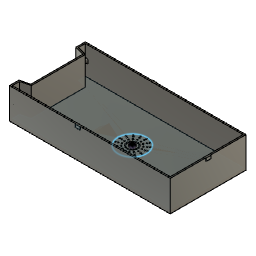
coolingpadbox v18 (Autodesk Fusion 360 design; units mm, degrees)
Autodesk Fusion 360 part; units mm, degrees
sketch "Sketch1" plane through (0, 0, 0) normal (1, 0, 0) x (0, 1, 0)
sketch "Sketch2" plane through (0, 0, 0) normal (0, 1, 0) x (1, 0, 0)
sketch "Sketch3" plane through (0, 0, 0) normal (0, 0, 1) x (1, 0, 0)
  line L0 (-89.6492, -40) -> (80, -40)
  line L1 (80, -40) -> (80, 40)
  line L2 (80, 40) -> (-89.6492, 40)
  line L3 (-89.6492, 40) -> (-89.6492, 30)
  line L4 (-89.6492, -40) -> (-89.6492, -30)
  line L5 (-89.6492, -40) -> (-79.6492, -40)
  line L6 (-79.6492, 27.5) -> (-79.6492, -27.5)
  line L7 (-79.6492, 27.5) -> (-89.6492, 30)
  line L8 (-89.6492, -30) -> (-79.6492, -27.5)
  constraint horizontal L0
  constraint perpendicular L0 L1
  constraint perpendicular L1 L2
  constraint coincident L0 L5.end
extrude "Extrude1" add sketch "Sketch3" along normal blind 2.5
sketch "Sketch4" plane through (0, 0, 2.5) normal (0, 0, 1) x (-1, 0, 0)
  line L0 (89.6492, 40) -> (-80, 40)
  line L1 (-80, 40) -> (-80, -40)
  line L2 (-80, -40) -> (89.6492, -40)
  line L3 (89.6492, -40) -> (89.6492, -30)
  line L4 (89.6492, -30) -> (79.6492, -27.5)
  line L5 (79.6492, -27.5) -> (79.6492, 27.5)
  line L6 (79.6492, 27.5) -> (89.6492, 30)
  line L7 (89.6492, 30) -> (89.6492, 40)
  line L8 (89.6492, -40) -> (-80, -40)
  line L9 (-80, -40) -> (-80, 40)
  line L10 (89.6492, 40) -> (-80, 40)
  line L11 (89.6492, 30) -> (89.6492, 40)
  line L12 (89.6492, 30) -> (79.6492, 27.5)
  line L13 (79.6492, 27.5) -> (79.6492, -27.5)
  line L14 (79.6492, -27.5) -> (89.6492, -30)
  line L15 (89.6492, -40) -> (89.6492, -30)
  line L16 (89.6492, -40) -> (89.6492, -38.5)
  line L17 (88.1492, -38.5) -> (-78.5, -38.5)
  line L18 (-80, -40) -> (-78.5, -40)
  line L19 (-78.5, -38.5) -> (-78.5, 38.5)
  line L20 (-80, 40) -> (-80, 38.5)
  line L21 (-78.5, 38.5) -> (88.1492, 38.5)
  line L22 (89.6492, 40) -> (88.1492, 40)
  line L23 (88.1492, 38.5) -> (88.1492, 31)
  line L24 (89.6492, 30) -> (89.6492, 31.375)
  line L25 (88.1492, 31) -> (78.1492, 28.5)
  line L26 (78.1492, -28.4841) -> (78.1492, 28.5)
  line L27 (89.6492, -40) -> (88.1492, -40)
  line L28 (88.1492, -31.1066) -> (88.1492, -38.5)
  line L29 (89.6492, -30) -> (89.6492, -31.5)
  line L30 (88.1492, -31.1066) -> (78.1492, -28.4841)
  dimension "d9" = 1.5
  dimension "d11" = 1.5
  constraint coincident L2.end L3.start
  constraint coincident L1.end L2.start
  constraint coincident L0.end L1.start
  constraint coincident L0.start L7.end
  constraint coincident L6.end L7.start
  constraint coincident L5.end L6.start
  constraint coincident L4.end L5.start
  constraint coincident L3.end L4.start
  constraint coincident L15 L16.end
  constraint perpendicular L1 L17
  constraint coincident L2 L18.end
  constraint perpendicular L9 L18
  constraint perpendicular L0 L19
  constraint coincident L1 L20.end
  constraint coincident L10 L22.end
  constraint perpendicular L0 L23
  constraint coincident L11 L24.end
  constraint parallel L6 L25
  constraint coincident L8 L27.end
  constraint perpendicular L2 L28
  constraint coincident L15 L29.end
  measures "d9" distance of L0.end L20.end
  measures "d11" distance of L0.start L22.end
extrude "Extrude2" add sketch "Sketch4" along normal blind 30
sketch "Sketch5" plane through (0, 0, 2.5) normal (0, 0, 1) x (-1, 0, 0)
  line L0 (88.1492, -31.1066) -> (78.1492, -28.4841)
  line L1 (78.1492, -28.4841) -> (78.1492, 28.5)
  line L2 (78.1492, 28.5) -> (88.1492, 31)
  line L3 (88.1492, 31) -> (88.1492, 38.5)
  line L4 (88.1492, 38.5) -> (-78.5, 38.5)
  line L5 (-78.5, 38.5) -> (-78.5, -38.5)
  line L6 (-78.5, -38.5) -> (88.1492, -38.5)
  line L7 (88.1492, -38.5) -> (88.1492, -31.1066)
sketch "Sketch6" plane through (0, 0, 32.5) normal (0, 0, 1) x (-1, 0, 0)
  line L0 (88.1492, -31.1066) -> (88.1492, -38.5)
  line L1 (88.1492, -38.5) -> (-78.5, -38.5)
  line L2 (-78.5, -38.5) -> (-78.5, 38.5)
  line L3 (-78.5, 38.5) -> (88.1492, 38.5)
  line L4 (88.1492, 38.5) -> (88.1492, 31)
  line L5 (88.1492, 31) -> (78.1492, 28.5)
  line L6 (78.1492, 28.5) -> (78.1492, -28.4841)
  line L7 (78.1492, -28.4841) -> (88.1492, -31.1066)
  line L8 (89.6492, 30) -> (89.6492, 40)
  line L9 (-80, 40) -> (-80, -40)
  line L10 (-80, -40) -> (89.6492, -40)
  line L11 (89.6492, -40) -> (89.6492, -30)
  line L12 (89.6492, -30) -> (79.6492, -27.5)
  line L13 (79.6492, -27.5) -> (79.6492, 27.5)
  line L14 (79.6492, 27.5) -> (89.6492, 30)
  line L15 (19.6492, 40) -> (14.6492, 40)
  line L16 (19.6492, -40) -> (14.6492, -40)
  line L17 (-80, 2.5) -> (-80, -2.5)
  line L18 (19.6492, 40) -> (14.6492, 40)
  line L19 (14.6492, 40) -> (14.6492, 40.5)
  line L20 (14.6492, 40.5) -> (19.6492, 40.5)
  line L21 (19.6492, 40.5) -> (19.6492, 40)
  line L22 (19.6492, -40) -> (14.6492, -40)
  line L23 (14.6492, -40) -> (14.6492, -40.5)
  line L24 (14.6492, -40.5) -> (19.6492, -40.5)
  line L25 (19.6492, -40.5) -> (19.6492, -40)
  line L26 (-80, -2.5) -> (-80.5, -2.5)
  line L27 (-80.5, -2.5) -> (-80.5, 2.5374)
  line L28 (-80.5, 2.5374) -> (-80, 2.5374)
  line L29 (-80, 2.5374) -> (-80, -2.5)
  dimension "d23" = 5
  dimension "d24" = 0.5
  dimension "d25" = 0.5
  dimension "d26" = 0.5
  constraint coincident L10 L16.start
  constraint coincident L10 L16.end
  constraint perpendicular L10 L17
  constraint horizontal L18
  constraint vertical L19
  constraint horizontal L20
  constraint vertical L21
  constraint horizontal L22
  constraint vertical L23
  constraint horizontal L24
  constraint vertical L25
  constraint horizontal L26
  constraint vertical L27
  constraint horizontal L28
  constraint vertical L29
  measures "d23" distance of L15.start L15.end
  measures "d24" distance of L15.start L20.end
  measures "d25" distance of L16.start L24.end
  measures "d26" distance of L17.end L26.end
extrude "Extrude3" add sketch "Sketch6" against normal blind 3 contours L9 L17 L26 L27 L28 L29 | L10 L16 L22 L23 L24 L25 | L15 L18 L19 L20 L21
sketch "Sketch7" plane through (0, -40.5, 0) normal (0, -1, 0) x (1, 0, 0)
  line L0 (-14.6492, 32.5) -> (-19.6492, 32.5)
  line L1 (-19.6492, 32.5) -> (-19.6492, 29.5)
  line L2 (-19.6492, 29.5) -> (-14.6492, 29.5)
  line L3 (-14.6492, 29.5) -> (-14.6492, 32.5)
hole "Hole1" at (-89.6492, -34.78, 16.965) direction (1, 0, 0) diameter 9 depth 4 tip angle 118
hole "Hole2" at (-89.6492, 34.6632, 17.2605) direction (1, 0, 0) diameter 9 depth 4 tip angle 118
sketch "Sketch8" plane through (0, 0, 0) normal (1, 0, 0) x (0, 1, 0)
sketch "Sketch9" plane through (0, 0, 2.5) normal (0, 0, 1) x (-1, 0, 0)
  circle A0 centre (0, 0) radius 15
  constraint coincident A0.centre origin
sketch "Sketch10" plane through (0, 0, 2.5) normal (0, 0, 1) x (-1, 0, 0)
  circle A0 centre (2, 0) radius 0.75
  circle A1 centre (5.3918, 0.0449) radius 0.75
  circle A2 centre (8.3496, -0.0273) radius 0.75
  circle A3 centre (11.3796, -0.0633) radius 0.75
  circle A4 centre (13.6527, -0.0633) radius 0.75
  circle A5 centre (2, 0) radius 1
  dimension "d36" = 1.5
  dimension "d37" = 1.5
  dimension "d38" = 1.5
  dimension "d39" = 1.5
  dimension "d40" = 1.5
  dimension "d47" = 2
  constraint concentric A0 A5
  measures "d36" diameter of A0
  measures "d37" diameter of A1
  measures "d38" diameter of A2
  measures "d39" diameter of A3
  measures "d40" diameter of A4
  measures "d47" diameter of A5
extrude "Extrude4" cut sketch "Sketch10" against normal blind 5 contours A0 | A1 | A2 | A3 | A4
pattern_circular "C-Pattern1" count 15 over 360 about axis through (0, 0, 2.5) along (0, 0, 1) of 4 faces at (-6.138, 0.0298, 1.6667) (-9.0959, 0.1019, 1.6667) (-12.1259, 0.138, 1.6667) (-14.399, 0.138, 1.6667)
pattern_circular "C-Pattern2" count 5 over 360 about axis through (0, 0, 2.5) along (0, 0, 1) of 1 faces at (-2.7463, 0.0747, 1.6667)
